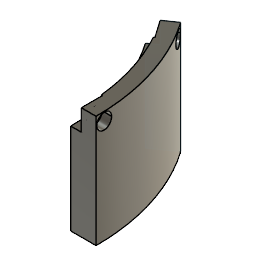
Access_Panel_2 (Autodesk Fusion 360 design; units mm, degrees)
Autodesk Fusion 360 part; units mm, degrees
sketch "Sketch1" plane through (0, 0, 0) normal (0, 0, 1) x (1, 0, 0)
  line L0 (90, 0) -> (102, 0)
  line L1 (73.7237, 51.6219) -> (83.5535, 58.5048)
  arc A0 (102, 0) -> (83.5535, 58.5048) centre (0, 0) ccw
  arc A1 (90, 0) -> (73.7237, 51.6219) centre (0, 0) ccw
  dimension "d1" = 204
  dimension "d2" = 180
  dimension "d3" = 145
  constraint coincident A0.centre A1.centre
  constraint horizontal L0
  measures "d1" diameter of A0
  measures "d2" diameter of A1
  measures "d3" angle of L0 L1
extrude "Extrude1" add sketch "Sketch1" along normal blind 43
sketch "Sketch2" plane through (0, 0, 43) normal (0, 0, 1) x (-1, 0, 0)
  arc A0 (-102, 0) -> (-83.5535, -58.5048) centre (0, 0) ccw
  line L0 (-83.5535, -58.5048) -> (-73.7237, -51.6219)
  arc A1 (-90, 0) -> (-73.7237, -51.6219) centre (0, 0) ccw
  line L1 (-90, 0) -> (-102, 0)
  circle A2 centre (0, 0) radius 102
  circle A3 centre (0, 0) radius 95
  line L2 (0, 0) -> (-83.5535, -58.5048)
  line L3 (0, 0) -> (-102, 0)
  dimension "d6" = 190
  constraint coincident A0.centre A1.centre
  constraint concentric A2 A3
  constraint coincident A0.end L0.start
  constraint coincident A0.start L1.end
  measures "d6" diameter of A3
extrude "Extrude2" add sketch "Sketch2" along normal blind 10 contours A0 L0 L1 A2 A3 L2 L3
sketch "Sketch3" plane through (0, 0, 0) normal (0, -1, 0) x (1, 0, 0)
  line L0 (90, 0) -> (102, 0)
  line L1 (102, 0) -> (102, 53)
  line L2 (102, 53) -> (95, 53)
  line L3 (95, 53) -> (95, 43)
  line L4 (95, 43) -> (90, 43)
  line L5 (90, 43) -> (90, 0)
  line L6 (90, 43) -> (95, 43)
  line L7 (95, 43) -> (95, 53)
  line L8 (95, 53) -> (90, 53)
  line L9 (90, 53) -> (90, 43)
  dimension "d9" = 5
  dimension "d10" = 10
  constraint coincident L4.end L5.start
  constraint perpendicular L3 L6
  constraint perpendicular L2 L7
  constraint perpendicular L3 L8
  constraint perpendicular L8 L9
  measures "d9" distance of L4.end L3.end
  measures "d10" distance of L3.end L2.end
revolve "Revolve1" cut sketch "Sketch3" angle 90 about axis through (95, 0, 53) along (1, 0, 0) contours L3 L4 L6 L7 L8 L9
sketch "Sketch4" plane through (0, 0, 0) normal (-0.573576, 0.819152, 0) x (-0.819152, -0.573576, 0)
  line L0 (-102, 0) -> (-90, 0)
  line L1 (-90, 0) -> (-90, 43)
  line L2 (-90, 43) -> (-95, 43)
  line L3 (-95, 43) -> (-95, 53)
  line L4 (-95, 53) -> (-102, 53)
  line L5 (-102, 53) -> (-102, 0)
sketch "Sketch5" plane through (0, 0, 0) normal (-0.573576, 0.819152, 0) x (-0.819152, -0.573576, 0)
  line L0 (-90, 43) -> (-95, 43)
  line L1 (-95, 43) -> (-95, 53)
  line L2 (-95, 53) -> (-90, 53)
  line L3 (-90, 53) -> (-90, 43)
  dimension "d12" = 5
  dimension "d13" = 10
  dimension "d14" = 5
  constraint horizontal L0
  constraint perpendicular L0 L1
  constraint perpendicular L1 L2
  measures "d12" distance of L0.start L0.end
  measures "d13" distance of L0.end L1.end
  measures "d14" distance of L1.end L2.end
revolve "Revolve2" cut sketch "Sketch5" angle 90 about axis through (77.8194, 54.4898, 53) along (-0.819152, -0.573576, 0)
sketch "Sketch6" plane through (77.8194, 54.4898, 0) normal (-0.819152, -0.573576, 0) x (0.573576, -0.819152, 0)
  line L0 (0, 53) -> (0, 43)
  arc A0 (0, 43) -> (10, 53) centre (0, 53) ccw
  line L1 (10, 53) -> (0, 53)
  line L2 (0, 53) -> (4, 53)
  line L3 (4, 53) -> (4, 49)
  circle A1 centre (4, 49) radius 2
  dimension "d16" = 4
  dimension "d17" = 4
  dimension "d18" = 4
  constraint coincident L0.start A0.centre
  constraint perpendicular L0 L2
  constraint perpendicular L1 L3
  constraint coincident L3.end A1.centre
  measures "d16" distance of L0.start L2.end
  measures "d17" distance of L2.end L3.end
  measures "d18" diameter of A1
extrude "Extrude3" cut sketch "Sketch6" against normal blind 10 contours A1
sketch "Sketch7" plane through (77.8194, 54.4898, 0) normal (-0.819152, -0.573576, 0) x (0.573576, -0.819152, 0)
  circle A0 centre (4, 49) radius 2
  line L0 (0, 53) -> (0, 43)
  arc A1 (0, 43) -> (10, 53) centre (0, 53) ccw
  line L1 (10, 53) -> (0, 53)
  circle A2 centre (4, 49) radius 3.65
  dimension "d21" = 7.3
  constraint concentric A0 A2
  measures "d21" diameter of A2
extrude "Extrude4" cut sketch "Sketch7" along normal blind 4.5 from the near side of the face at (96.6345, 32.6463, 17.6667) contours A2
sketch "Sketch8" plane through (95, 0, 0) normal (-1, 0, 0) x (0, -1, 0)
  line L0 (0, 43) -> (0, 53)
  line L1 (0, 53) -> (-10, 53)
  arc A0 (-10, 53) -> (0, 43) centre (0, 53) ccw
  line L2 (0, 53) -> (-4, 53)
  line L3 (-4, 53) -> (-4, 49)
  circle A1 centre (-4, 49) radius 2
  dimension "d24" = 4
  dimension "d25" = 4
  dimension "d26" = 4
  constraint coincident L0.end L1.start
  constraint perpendicular L0 L2
  constraint perpendicular L1 L3
  constraint coincident L3.end A1.centre
  measures "d24" distance of L0.end L2.end
  measures "d25" distance of L2.end L3.end
  measures "d26" diameter of A1
extrude "Extrude5" cut sketch "Sketch8" against normal blind 10 contours A1
sketch "Sketch9" plane through (95, 0, 0) normal (-1, 0, 0) x (0, -1, 0)
  circle A0 centre (-4, 49) radius 2
  line L0 (0, 43) -> (0, 53)
  line L1 (0, 53) -> (-10, 53)
  arc A1 (-10, 53) -> (0, 43) centre (0, 53) ccw
  circle A2 centre (-4, 49) radius 3.65
  dimension "d29" = 7.3
  constraint concentric A0 A2
  measures "d29" diameter of A2
extrude "Extrude6" cut sketch "Sketch9" along normal blind 4.5 from the near side of the face at (96.6345, 32.6463, 17.6667) contours A2
